Autodesk Fusion 360 part; units mm, degrees
(part 29 of 40)
  spline S86 degree 5 poles (187.9372, 93.9655) (187.9249, 93.9372) (187.9012, 93.8802) (187.868, 93.7938) (187.8281, 93.6771) (187.7842, 93.5289) (187.7447, 93.3792) (187.7079, 93.2286) (187.6725, 93.0774) (187.638, 92.9259) (187.6046, 92.774) (187.5726, 92.6217) (187.5424, 92.4688) (187.5144, 92.3152) (187.4885, 92.1609) (187.4646, 92.006) (187.4423, 91.8506) (187.4215, 91.6948) (187.4019, 91.5386) (187.3835, 91.3821) (187.3662, 91.2253) (187.3502, 91.0682) (187.3355, 90.9107) (187.3222, 90.7529) (187.3102, 90.5947) (187.2995, 90.4362) (187.29, 90.2774) (187.2816, 90.1183) (187.2743, 89.9589) (187.2682, 89.7993) (187.2631, 89.6395) (187.2591, 89.4794) (187.2563, 89.3191) (187.2544, 89.1585) (187.2537, 88.9977) (187.254, 88.8367) (187.2554, 88.6755) (187.2578, 88.5141) (187.2612, 88.3525) (187.2655, 88.1907) (187.2709, 88.0288) (187.2772, 87.8666) (187.2845, 87.7043) (187.2928, 87.5419) (187.302, 87.3793) (187.3121, 87.2165) (187.3232, 87.0536) (187.3353, 86.8905) (187.3482, 86.7273) (187.362, 86.564) (187.3768, 86.4005) (187.3924, 86.2369) (187.409, 86.0732) (187.4264, 85.9094) (187.4447, 85.7455) (187.4639, 85.5815) (187.484, 85.4174) (187.5049, 85.2532) (187.5266, 85.0889) (187.5492, 84.9245) (187.5727, 84.76) (187.597, 84.5954) (187.6222, 84.4308) (187.6481, 84.266) (187.6749, 84.1013) (187.7026, 83.9364) (187.731, 83.7715) (187.7602, 83.6065) (187.7903, 83.4415) (187.8212, 83.2764) (187.8528, 83.1113) (187.8788, 82.9792) (187.8986, 82.8801) (187.912, 82.814) (187.9188, 82.7809) knots 0 0 0 0 0 0 0.01428571 0.02857143 0.04285714 0.05714286 0.07142857 0.08571429 0.1 0.11428571 0.12857143 0.14285714 0.15714286 0.17142857 0.18571429 0.2 0.21428571 0.22857143 0.24285714 0.25714286 0.27142857 0.28571429 0.3 0.31428571 0.32857143 0.34285714 0.35714286 0.37142857 0.38571429 0.4 0.41428571 0.42857143 0.44285714 0.45714286 0.47142857 0.48571429 0.5 0.51428571 0.52857143 0.54285714 0.55714286 0.57142857 0.58571429 0.6 0.61428571 0.62857143 0.64285714 0.65714286 0.67142857 0.68571429 0.7 0.71428571 0.72857143 0.74285714 0.75714286 0.77142857 0.78571429 0.8 0.81428571 0.82857143 0.84285714 0.85714286 0.87142857 0.88571429 0.9 0.91428571 0.92857143 0.94285714 0.95714286 0.97142857 0.98571429 1 1 1 1 1 1
  line L6451 (187.9372, 93.9655) -> (187.9249, 93.9372) construction
  line L6452 (187.9249, 93.9372) -> (187.9012, 93.8802) construction
  line L6453 (187.9012, 93.8802) -> (187.868, 93.7938) construction
  line L6454 (187.868, 93.7938) -> (187.8281, 93.6771) construction
  line L6455 (187.8281, 93.6771) -> (187.7842, 93.5289) construction
  line L6456 (187.7842, 93.5289) -> (187.7447, 93.3792) construction
  line L6457 (187.7447, 93.3792) -> (187.7079, 93.2286) construction
  line L6458 (187.7079, 93.2286) -> (187.6725, 93.0774) construction
  line L6459 (187.6725, 93.0774) -> (187.638, 92.9259) construction
  line L6460 (187.638, 92.9259) -> (187.6046, 92.774) construction
  line L6461 (187.6046, 92.774) -> (187.5726, 92.6217) construction
  line L6462 (187.5726, 92.6217) -> (187.5424, 92.4688) construction
  line L6463 (187.5424, 92.4688) -> (187.5144, 92.3152) construction
  line L6464 (187.5144, 92.3152) -> (187.4885, 92.1609) construction
  line L6465 (187.4885, 92.1609) -> (187.4646, 92.006) construction
  line L6466 (187.4646, 92.006) -> (187.4423, 91.8506) construction
  line L6467 (187.4423, 91.8506) -> (187.4215, 91.6948) construction
  line L6468 (187.4215, 91.6948) -> (187.4019, 91.5386) construction
  line L6469 (187.4019, 91.5386) -> (187.3835, 91.3821) construction
  line L6470 (187.3835, 91.3821) -> (187.3662, 91.2253) construction
  line L6471 (187.3662, 91.2253) -> (187.3502, 91.0682) construction
  line L6472 (187.3502, 91.0682) -> (187.3355, 90.9107) construction
  line L6473 (187.3355, 90.9107) -> (187.3222, 90.7529) construction
  line L6474 (187.3222, 90.7529) -> (187.3102, 90.5947) construction
  line L6475 (187.3102, 90.5947) -> (187.2995, 90.4362) construction
  line L6476 (187.2995, 90.4362) -> (187.29, 90.2774) construction
  line L6477 (187.29, 90.2774) -> (187.2816, 90.1183) construction
  line L6478 (187.2816, 90.1183) -> (187.2743, 89.9589) construction
  line L6479 (187.2743, 89.9589) -> (187.2682, 89.7993) construction
  line L6480 (187.2682, 89.7993) -> (187.2631, 89.6395) construction
  line L6481 (187.2631, 89.6395) -> (187.2591, 89.4794) construction
  line L6482 (187.2591, 89.4794) -> (187.2563, 89.3191) construction
  line L6483 (187.2563, 89.3191) -> (187.2544, 89.1585) construction
  line L6484 (187.2544, 89.1585) -> (187.2537, 88.9977) construction
  line L6485 (187.2537, 88.9977) -> (187.254, 88.8367) construction
  line L6486 (187.254, 88.8367) -> (187.2554, 88.6755) construction
  line L6487 (187.2554, 88.6755) -> (187.2578, 88.5141) construction
  line L6488 (187.2578, 88.5141) -> (187.2612, 88.3525) construction
  line L6489 (187.2612, 88.3525) -> (187.2655, 88.1907) construction
  line L6490 (187.2655, 88.1907) -> (187.2709, 88.0288) construction
  line L6491 (187.2709, 88.0288) -> (187.2772, 87.8666) construction
  line L6492 (187.2772, 87.8666) -> (187.2845, 87.7043) construction
  line L6493 (187.2845, 87.7043) -> (187.2928, 87.5419) construction
  line L6494 (187.2928, 87.5419) -> (187.302, 87.3793) construction
  line L6495 (187.302, 87.3793) -> (187.3121, 87.2165) construction
  line L6496 (187.3121, 87.2165) -> (187.3232, 87.0536) construction
  line L6497 (187.3232, 87.0536) -> (187.3353, 86.8905) construction
  line L6498 (187.3353, 86.8905) -> (187.3482, 86.7273) construction
  line L6499 (187.3482, 86.7273) -> (187.362, 86.564) construction
  line L6500 (187.362, 86.564) -> (187.3768, 86.4005) construction
  line L6501 (187.3768, 86.4005) -> (187.3924, 86.2369) construction
  line L6502 (187.3924, 86.2369) -> (187.409, 86.0732) construction
  line L6503 (187.409, 86.0732) -> (187.4264, 85.9094) construction
  line L6504 (187.4264, 85.9094) -> (187.4447, 85.7455) construction
  line L6505 (187.4447, 85.7455) -> (187.4639, 85.5815) construction
  line L6506 (187.4639, 85.5815) -> (187.484, 85.4174) construction
  line L6507 (187.484, 85.4174) -> (187.5049, 85.2532) construction
  line L6508 (187.5049, 85.2532) -> (187.5266, 85.0889) construction
  line L6509 (187.5266, 85.0889) -> (187.5492, 84.9245) construction
  line L6510 (187.5492, 84.9245) -> (187.5727, 84.76) construction
  line L6511 (187.5727, 84.76) -> (187.597, 84.5954) construction
  line L6512 (187.597, 84.5954) -> (187.6222, 84.4308) construction
  line L6513 (187.6222, 84.4308) -> (187.6481, 84.266) construction
  line L6514 (187.6481, 84.266) -> (187.6749, 84.1013) construction
  line L6515 (187.6749, 84.1013) -> (187.7026, 83.9364) construction
  line L6516 (187.7026, 83.9364) -> (187.731, 83.7715) construction
  line L6517 (187.731, 83.7715) -> (187.7602, 83.6065) construction
  line L6518 (187.7602, 83.6065) -> (187.7903, 83.4415) construction
  line L6519 (187.7903, 83.4415) -> (187.8212, 83.2764) construction
  line L6520 (187.8212, 83.2764) -> (187.8528, 83.1113) construction
  line L6521 (187.8528, 83.1113) -> (187.8788, 82.9792) construction
  line L6522 (187.8788, 82.9792) -> (187.8986, 82.8801) construction
  line L6523 (187.8986, 82.8801) -> (187.912, 82.814) construction
  line L6524 (187.912, 82.814) -> (187.9188, 82.7809) construction
  line L6525 (152.9878, 155.5428) -> (151.3635, 155.6951)
  line L6526 (199.127, 207.9623) -> (198.7698, 209.5542)
  line L6527 (225.137, 207.9623) -> (225.4942, 209.5542)
  line L6528 (217.6748, 209.1442) -> (217.8271, 210.7685)
  line L6529 (251.3803, 194.5906) -> (252.4583, 195.8153)
  line L6530 (271.2762, 155.5428) -> (272.9005, 155.6951)
  line L6531 (172.8837, 194.5906) -> (171.8057, 195.8153)
  line L6532 (181.8522, 201.1066) -> (181.0205, 202.5103)
  line L6533 (157.5954, 173.5481) -> (156.0975, 174.1948)
  line L6534 (167.5414, 189.2483) -> (166.3167, 190.3263)
  spline S87 degree 5 poles (166.3167, 109.6737) (166.2935, 109.6533) (166.2466, 109.6132) (166.1747, 109.5549) (166.076, 109.4808) (165.9487, 109.3934) (165.8185, 109.3096) (165.6866, 109.228) (165.5538, 109.1476) (165.4203, 109.068) (165.2862, 108.9893) (165.1513, 108.9117) (165.0152, 108.8358) (164.8777, 108.7617) (164.739, 108.6894) (164.5991, 108.6187) (164.4582, 108.5496) (164.3164, 108.4816) (164.1739, 108.4147) (164.0308, 108.3488) (163.887, 108.284) (163.7425, 108.2202) (163.5973, 108.1576) (163.4513, 108.0961) (163.3046, 108.0358) (163.1571, 107.9766) (163.009, 107.9185) (162.8603, 107.8614) (162.711, 107.8053) (162.5611, 107.7501) (162.4106, 107.6959) (162.2596, 107.6426) (162.108, 107.5903) (161.9559, 107.539) (161.8032, 107.4886) (161.65, 107.4392) (161.4962, 107.3906) (161.342, 107.343) (161.1873, 107.2963) (161.0321, 107.2505) (160.8764, 107.2055) (160.7202, 107.1614) (160.5636, 107.1182) (160.4065, 107.0759) (160.249, 107.0344) (160.0911, 106.9937) (159.9327, 106.9539) (159.7739, 106.915) (159.6147, 106.8769) (159.4551, 106.8396) (159.2951, 106.8031) (159.1347, 106.7674) (158.9739, 106.7326) (158.8127, 106.6985) (158.6511, 106.6653) (158.4892, 106.6328) (158.3269, 106.6012) (158.1643, 106.5703) (158.0013, 106.5403) (157.838, 106.511) (157.6743, 106.4825) (157.5103, 106.4547) (157.3459, 106.4277) (157.1812, 106.4016) (157.0162, 106.3761) (156.8509, 106.3514) (156.6853, 106.3275) (156.5194, 106.3044) (156.3531, 106.282) (156.1866, 106.2603) (156.0198, 106.2394) (155.8861, 106.2233) (155.7857, 106.2115) (155.7187, 106.2038) (155.6851, 106.2) knots 0 0 0 0 0 0 0.01428571 0.02857143 0.04285714 0.05714286 0.07142857 0.08571429 0.1 0.11428571 0.12857143 0.14285714 0.15714286 0.17142857 0.18571429 0.2 0.21428571 0.22857143 0.24285714 0.25714286 0.27142857 0.28571429 0.3 0.31428571 0.32857143 0.34285714 0.35714286 0.37142857 0.38571429 0.4 0.41428571 0.42857143 0.44285714 0.45714286 0.47142857 0.48571429 0.5 0.51428571 0.52857143 0.54285714 0.55714286 0.57142857 0.58571429 0.6 0.61428571 0.62857143 0.64285714 0.65714286 0.67142857 0.68571429 0.7 0.71428571 0.72857143 0.74285714 0.75714286 0.77142857 0.78571429 0.8 0.81428571 0.82857143 0.84285714 0.85714286 0.87142857 0.88571429 0.9 0.91428571 0.92857143 0.94285714 0.95714286 0.97142857 0.98571429 1 1 1 1 1 1
  line L6535 (166.3167, 109.6737) -> (166.2935, 109.6533) construction
  line L6536 (166.2935, 109.6533) -> (166.2466, 109.6132) construction
  line L6537 (166.2466, 109.6132) -> (166.1747, 109.5549) construction
  line L6538 (166.1747, 109.5549) -> (166.076, 109.4808) construction
  line L6539 (166.076, 109.4808) -> (165.9487, 109.3934) construction
  line L6540 (165.9487, 109.3934) -> (165.8185, 109.3096) construction
  line L6541 (165.8185, 109.3096) -> (165.6866, 109.228) construction
  line L6542 (165.6866, 109.228) -> (165.5538, 109.1476) construction
  line L6543 (165.5538, 109.1476) -> (165.4203, 109.068) construction
  line L6544 (165.4203, 109.068) -> (165.2862, 108.9893) construction
  line L6545 (165.2862, 108.9893) -> (165.1513, 108.9117) construction
  line L6546 (165.1513, 108.9117) -> (165.0152, 108.8358) construction
  line L6547 (165.0152, 108.8358) -> (164.8777, 108.7617) construction
  line L6548 (164.8777, 108.7617) -> (164.739, 108.6894) construction
  line L6549 (164.739, 108.6894) -> (164.5991, 108.6187) construction
  line L6550 (164.5991, 108.6187) -> (164.4582, 108.5496) construction
  line L6551 (164.4582, 108.5496) -> (164.3164, 108.4816) construction
  line L6552 (164.3164, 108.4816) -> (164.1739, 108.4147) construction
  line L6553 (164.1739, 108.4147) -> (164.0308, 108.3488) construction
  line L6554 (164.0308, 108.3488) -> (163.887, 108.284) construction
  line L6555 (163.887, 108.284) -> (163.7425, 108.2202) construction
  line L6556 (163.7425, 108.2202) -> (163.5973, 108.1576) construction
  line L6557 (163.5973, 108.1576) -> (163.4513, 108.0961) construction
  line L6558 (163.4513, 108.0961) -> (163.3046, 108.0358) construction
  line L6559 (163.3046, 108.0358) -> (163.1571, 107.9766) construction
  line L6560 (163.1571, 107.9766) -> (163.009, 107.9185) construction
  line L6561 (163.009, 107.9185) -> (162.8603, 107.8614) construction
  line L6562 (162.8603, 107.8614) -> (162.711, 107.8053) construction
  line L6563 (162.711, 107.8053) -> (162.5611, 107.7501) construction
  line L6564 (162.5611, 107.7501) -> (162.4106, 107.6959) construction
  line L6565 (162.4106, 107.6959) -> (162.2596, 107.6426) construction
  line L6566 (162.2596, 107.6426) -> (162.108, 107.5903) construction
  line L6567 (162.108, 107.5903) -> (161.9559, 107.539) construction
  line L6568 (161.9559, 107.539) -> (161.8032, 107.4886) construction
  line L6569 (161.8032, 107.4886) -> (161.65, 107.4392) construction
  line L6570 (161.65, 107.4392) -> (161.4962, 107.3906) construction
  line L6571 (161.4962, 107.3906) -> (161.342, 107.343) construction
  line L6572 (161.342, 107.343) -> (161.1873, 107.2963) construction
  line L6573 (161.1873, 107.2963) -> (161.0321, 107.2505) construction
  line L6574 (161.0321, 107.2505) -> (160.8764, 107.2055) construction
  line L6575 (160.8764, 107.2055) -> (160.7202, 107.1614) construction
  line L6576 (160.7202, 107.1614) -> (160.5636, 107.1182) construction
  line L6577 (160.5636, 107.1182) -> (160.4065, 107.0759) construction
  line L6578 (160.4065, 107.0759) -> (160.249, 107.0344) construction
  line L6579 (160.249, 107.0344) -> (160.0911, 106.9937) construction
  line L6580 (160.0911, 106.9937) -> (159.9327, 106.9539) construction
  line L6581 (159.9327, 106.9539) -> (159.7739, 106.915) construction
  line L6582 (159.7739, 106.915) -> (159.6147, 106.8769) construction
  line L6583 (159.6147, 106.8769) -> (159.4551, 106.8396) construction
  line L6584 (159.4551, 106.8396) -> (159.2951, 106.8031) construction
  line L6585 (159.2951, 106.8031) -> (159.1347, 106.7674) construction
  line L6586 (159.1347, 106.7674) -> (158.9739, 106.7326) construction
  line L6587 (158.9739, 106.7326) -> (158.8127, 106.6985) construction
  line L6588 (158.8127, 106.6985) -> (158.6511, 106.6653) construction
  line L6589 (158.6511, 106.6653) -> (158.4892, 106.6328) construction
  line L6590 (158.4892, 106.6328) -> (158.3269, 106.6012) construction
  line L6591 (158.3269, 106.6012) -> (158.1643, 106.5703) construction
  line L6592 (158.1643, 106.5703) -> (158.0013, 106.5403) construction
  line L6593 (158.0013, 106.5403) -> (157.838, 106.511) construction
  line L6594 (157.838, 106.511) -> (157.6743, 106.4825) construction
  line L6595 (157.6743, 106.4825) -> (157.5103, 106.4547) construction
  line L6596 (157.5103, 106.4547) -> (157.3459, 106.4277) construction
  line L6597 (157.3459, 106.4277) -> (157.1812, 106.4016) construction
  line L6598 (157.1812, 106.4016) -> (157.0162, 106.3761) construction
  line L6599 (157.0162, 106.3761) -> (156.8509, 106.3514) construction
  line L6600 (156.8509, 106.3514) -> (156.6853, 106.3275) construction
  line L6601 (156.6853, 106.3275) -> (156.5194, 106.3044) construction
  line L6602 (156.5194, 106.3044) -> (156.3531, 106.282) construction
  line L6603 (156.3531, 106.282) -> (156.1866, 106.2603) construction
  line L6604 (156.1866, 106.2603) -> (156.0198, 106.2394) construction
  line L6605 (156.0198, 106.2394) -> (155.8861, 106.2233) construction
  line L6606 (155.8861, 106.2233) -> (155.7857, 106.2115) construction
  line L6607 (155.7857, 106.2115) -> (155.7187, 106.2038) construction
  line L6608 (155.7187, 106.2038) -> (155.6851, 106.2) construction
  arc A175 (236.3452, 217.2191) -> (232.0535, 218.6136) centre (212.132, 150) ccw
  spline S88 degree 5 poles (236.3268, 206.0345) (236.3391, 206.0628) (236.3628, 206.1198) (236.396, 206.2062) (236.4359, 206.3229) (236.4798, 206.4711) (236.5193, 206.6208) (236.5561, 206.7714) (236.5915, 206.9226) (236.626, 207.0741) (236.6594, 207.226) (236.6914, 207.3783) (236.7216, 207.5312) (236.7496, 207.6848) (236.7755, 207.8391) (236.7994, 207.994) (236.8217, 208.1494) (236.8425, 208.3052) (236.8621, 208.4614) (236.8805, 208.6179) (236.8978, 208.7747) (236.9138, 208.9318) (236.9285, 209.0893) (236.9418, 209.2471) (236.9538, 209.4053) (236.9645, 209.5638) (236.974, 209.7226) (236.9824, 209.8817) (236.9897, 210.0411) (236.9958, 210.2007) (237.0009, 210.3605) (237.0049, 210.5206) (237.0077, 210.6809) (237.0096, 210.8415) (237.0103, 211.0023) (237.01, 211.1633) (237.0086, 211.3245) (237.0062, 211.4859) (237.0028, 211.6475) (236.9985, 211.8093) (236.9931, 211.9712) (236.9868, 212.1334) (236.9795, 212.2957) (236.9712, 212.4581) (236.962, 212.6207) (236.9519, 212.7835) (236.9408, 212.9464) (236.9287, 213.1095) (236.9158, 213.2727) (236.902, 213.436) (236.8872, 213.5995) (236.8716, 213.7631) (236.855, 213.9268) (236.8376, 214.0906) (236.8193, 214.2545) (236.8001, 214.4185) (236.78, 214.5826) (236.7591, 214.7468) (236.7374, 214.9111) (236.7148, 215.0755) (236.6913, 215.24) (236.667, 215.4046) (236.6418, 215.5692) (236.6159, 215.734) (236.5891, 215.8987) (236.5614, 216.0636) (236.533, 216.2285) (236.5038, 216.3935) (236.4737, 216.5585) (236.4428, 216.7236) (236.4112, 216.8887) (236.3852, 217.0208) (236.3654, 217.1199) (236.352, 217.186) (236.3452, 217.2191) knots 0 0 0 0 0 0 0.01428571 0.02857143 0.04285714 0.05714286 0.07142857 0.08571429 0.1 0.11428571 0.12857143 0.14285714 0.15714286 0.17142857 0.18571429 0.2 0.21428571 0.22857143 0.24285714 0.25714286 0.27142857 0.28571429 0.3 0.31428571 0.32857143 0.34285714 0.35714286 0.37142857 0.38571429 0.4 0.41428571 0.42857143 0.44285714 0.45714286 0.47142857 0.48571429 0.5 0.51428571 0.52857143 0.54285714 0.55714286 0.57142857 0.58571429 0.6 0.61428571 0.62857143 0.64285714 0.65714286 0.67142857 0.68571429 0.7 0.71428571 0.72857143 0.74285714 0.75714286 0.77142857 0.78571429 0.8 0.81428571 0.82857143 0.84285714 0.85714286 0.87142857 0.88571429 0.9 0.91428571 0.92857143 0.94285714 0.95714286 0.97142857 0.98571429 1 1 1 1 1 1
  line L6609 (236.3268, 206.0345) -> (236.3391, 206.0628) construction
  line L6610 (236.3391, 206.0628) -> (236.3628, 206.1198) construction
  line L6611 (236.3628, 206.1198) -> (236.396, 206.2062) construction
  line L6612 (236.396, 206.2062) -> (236.4359, 206.3229) construction
  line L6613 (236.4359, 206.3229) -> (236.4798, 206.4711) construction
  line L6614 (236.4798, 206.4711) -> (236.5193, 206.6208) construction
  line L6615 (236.5193, 206.6208) -> (236.5561, 206.7714) construction
  line L6616 (236.5561, 206.7714) -> (236.5915, 206.9226) construction
  line L6617 (236.5915, 206.9226) -> (236.626, 207.0741) construction
  line L6618 (236.626, 207.0741) -> (236.6594, 207.226) construction
  line L6619 (236.6594, 207.226) -> (236.6914, 207.3783) construction
  line L6620 (236.6914, 207.3783) -> (236.7216, 207.5312) construction
  line L6621 (236.7216, 207.5312) -> (236.7496, 207.6848) construction
  line L6622 (236.7496, 207.6848) -> (236.7755, 207.8391) construction
  line L6623 (236.7755, 207.8391) -> (236.7994, 207.994) construction
  line L6624 (236.7994, 207.994) -> (236.8217, 208.1494) construction
  line L6625 (236.8217, 208.1494) -> (236.8425, 208.3052) construction
  line L6626 (236.8425, 208.3052) -> (236.8621, 208.4614) construction
  line L6627 (236.8621, 208.4614) -> (236.8805, 208.6179) construction
  line L6628 (236.8805, 208.6179) -> (236.8978, 208.7747) construction
  line L6629 (236.8978, 208.7747) -> (236.9138, 208.9318) construction
  line L6630 (236.9138, 208.9318) -> (236.9285, 209.0893) construction
  line L6631 (236.9285, 209.0893) -> (236.9418, 209.2471) construction
  line L6632 (236.9418, 209.2471) -> (236.9538, 209.4053) construction
  line L6633 (236.9538, 209.4053) -> (236.9645, 209.5638) construction
  line L6634 (236.9645, 209.5638) -> (236.974, 209.7226) construction
  line L6635 (236.974, 209.7226) -> (236.9824, 209.8817) construction
  line L6636 (236.9824, 209.8817) -> (236.9897, 210.0411) construction
  line L6637 (236.9897, 210.0411) -> (236.9958, 210.2007) construction
  line L6638 (236.9958, 210.2007) -> (237.0009, 210.3605) construction
  line L6639 (237.0009, 210.3605) -> (237.0049, 210.5206) construction
  line L6640 (237.0049, 210.5206) -> (237.0077, 210.6809) construction
  line L6641 (237.0077, 210.6809) -> (237.0096, 210.8415) construction
  line L6642 (237.0096, 210.8415) -> (237.0103, 211.0023) construction
  line L6643 (237.0103, 211.0023) -> (237.01, 211.1633) construction
  line L6644 (237.01, 211.1633) -> (237.0086, 211.3245) construction
  line L6645 (237.0086, 211.3245) -> (237.0062, 211.4859) construction
  line L6646 (237.0062, 211.4859) -> (237.0028, 211.6475) construction
  line L6647 (237.0028, 211.6475) -> (236.9985, 211.8093) construction
  line L6648 (236.9985, 211.8093) -> (236.9931, 211.9712) construction
  line L6649 (236.9931, 211.9712) -> (236.9868, 212.1334) construction
  line L6650 (236.9868, 212.1334) -> (236.9795, 212.2957) construction
  line L6651 (236.9795, 212.2957) -> (236.9712, 212.4581) construction
  line L6652 (236.9712, 212.4581) -> (236.962, 212.6207) construction
  line L6653 (236.962, 212.6207) -> (236.9519, 212.7835) construction
  line L6654 (236.9519, 212.7835) -> (236.9408, 212.9464) construction
  line L6655 (236.9408, 212.9464) -> (236.9287, 213.1095) construction
  line L6656 (236.9287, 213.1095) -> (236.9158, 213.2727) construction
  line L6657 (236.9158, 213.2727) -> (236.902, 213.436) construction
  line L6658 (236.902, 213.436) -> (236.8872, 213.5995) construction
  line L6659 (236.8872, 213.5995) -> (236.8716, 213.7631) construction
  line L6660 (236.8716, 213.7631) -> (236.855, 213.9268) construction
  line L6661 (236.855, 213.9268) -> (236.8376, 214.0906) construction
  line L6662 (236.8376, 214.0906) -> (236.8193, 214.2545) construction
  line L6663 (236.8193, 214.2545) -> (236.8001, 214.4185) construction
  line L6664 (236.8001, 214.4185) -> (236.78, 214.5826) construction
  line L6665 (236.78, 214.5826) -> (236.7591, 214.7468) construction
  line L6666 (236.7591, 214.7468) -> (236.7374, 214.9111) construction
  line L6667 (236.7374, 214.9111) -> (236.7148, 215.0755) construction
  line L6668 (236.7148, 215.0755) -> (236.6913, 215.24) construction
  line L6669 (236.6913, 215.24) -> (236.667, 215.4046) construction
  line L6670 (236.667, 215.4046) -> (236.6418, 215.5692) construction
  line L6671 (236.6418, 215.5692) -> (236.6159, 215.734) construction
  line L6672 (236.6159, 215.734) -> (236.5891, 215.8987) construction
  line L6673 (236.5891, 215.8987) -> (236.5614, 216.0636) construction
  line L6674 (236.5614, 216.0636) -> (236.533, 216.2285) construction
  line L6675 (236.533, 216.2285) -> (236.5038, 216.3935) construction
  line L6676 (236.5038, 216.3935) -> (236.4737, 216.5585) construction
  line L6677 (236.4737, 216.5585) -> (236.4428, 216.7236) construction
  line L6678 (236.4428, 216.7236) -> (236.4112, 216.8887) construction
  line L6679 (236.4112, 216.8887) -> (236.3852, 217.0208) construction
  line L6680 (236.3852, 217.0208) -> (236.3654, 217.1199) construction
  line L6681 (236.3654, 217.1199) -> (236.352, 217.186) construction
  line L6682 (236.352, 217.186) -> (236.3452, 217.2191) construction
  arc A176 (239.7302, 200.3721) -> (242.4118, 201.1066) centre (240.6912, 202.1261) ccw
  spline S89 degree 5 poles (271.6862, 136.6378) (271.7163, 136.631) (271.7764, 136.6167) (271.8658, 136.5929) (271.9837, 136.5565) (272.1293, 136.5049) (272.2736, 136.4489) (272.4172, 136.3901) (272.5603, 136.3299) (272.7031, 136.2687) (272.8456, 136.2065) (272.9877, 136.1429) (273.1291, 136.0774) (273.2699, 136.0098) (273.4099, 135.94) (273.5493, 135.8684) (273.6881, 135.795) (273.8264, 135.7203) (273.9642, 135.6443) (274.1017, 135.5673) (274.2387, 135.4891) (274.3752, 135.4096) (274.5112, 135.3289) (274.6468, 135.247) (274.7818, 135.1637) (274.9163, 135.0792) (275.0504, 134.9936) (275.184, 134.9068) (275.3172, 134.819) (275.45, 134.7302) (275.5823, 134.6403) (275.7141, 134.5494) (275.8455, 134.4575) (275.9765, 134.3646) (276.107, 134.2707) (276.237, 134.1758) (276.3666, 134.08) (276.4958, 133.9832) (276.6246, 133.8854) (276.7529, 133.7868) (276.8808, 133.6873) (277.0082, 133.5869) (277.1352, 133.4856) (277.2618, 133.3834) (277.388, 133.2804) (277.5137, 133.1765) (277.639, 133.0717) (277.7638, 132.9662) (277.8882, 132.8598) (278.0122, 132.7526) (278.1358, 132.6445) (278.2589, 132.5357) (278.3817, 132.4261) (278.5039, 132.3158) (278.6258, 132.2046) (278.7472, 132.0927) (278.8682, 131.98) (278.9888, 131.8665) (279.1089, 131.7523) (279.2286, 131.6374) (279.3479, 131.5218) (279.4667, 131.4054) (279.5851, 131.2882) (279.7031, 131.1704) (279.8207, 131.0519) (279.9378, 130.9326) (280.0545, 130.8127) (280.1708, 130.6921) (280.2866, 130.5707) (280.402, 130.4488) (280.517, 130.3261) (280.6087, 130.2274) (280.6772, 130.1531) (280.7228, 130.1034) (280.7456, 130.0785) knots 0 0 0 0 0 0 0.01428571 0.02857143 0.04285714 0.05714286 0.07142857 0.08571429 0.1 0.11428571 0.12857143 0.14285714 0.15714286 0.17142857 0.18571429 0.2 0.21428571 0.22857143 0.24285714 0.25714286 0.27142857 0.28571429 0.3 0.31428571 0.32857143 0.34285714 0.35714286 0.37142857 0.38571429 0.4 0.41428571 0.42857143 0.44285714 0.45714286 0.47142857 0.48571429 0.5 0.51428571 0.52857143 0.54285714 0.55714286 0.57142857 0.58571429 0.6 0.61428571 0.62857143 0.64285714 0.65714286 0.67142857 0.68571429 0.7 0.71428571 0.72857143 0.74285714 0.75714286 0.77142857 0.78571429 0.8 0.81428571 0.82857143 0.84285714 0.85714286 0.87142857 0.88571429 0.9 0.91428571 0.92857143 0.94285714 0.95714286 0.97142857 0.98571429 1 1 1 1 1 1
  line L6683 (271.6862, 136.6378) -> (271.7163, 136.631) construction
  line L6684 (271.7163, 136.631) -> (271.7764, 136.6167) construction
  line L6685 (271.7764, 136.6167) -> (271.8658, 136.5929) construction
  line L6686 (271.8658, 136.5929) -> (271.9837, 136.5565) construction
  line L6687 (271.9837, 136.5565) -> (272.1293, 136.5049) construction
  line L6688 (272.1293, 136.5049) -> (272.2736, 136.4489) construction
  line L6689 (272.2736, 136.4489) -> (272.4172, 136.3901) construction
  line L6690 (272.4172, 136.3901) -> (272.5603, 136.3299) construction
  line L6691 (272.5603, 136.3299) -> (272.7031, 136.2687) construction
  line L6692 (272.7031, 136.2687) -> (272.8456, 136.2065) construction
  line L6693 (272.8456, 136.2065) -> (272.9877, 136.1429) construction
  line L6694 (272.9877, 136.1429) -> (273.1291, 136.0774) construction
  line L6695 (273.1291, 136.0774) -> (273.2699, 136.0098) construction
  line L6696 (273.2699, 136.0098) -> (273.4099, 135.94) construction
  line L6697 (273.4099, 135.94) -> (273.5493, 135.8684) construction
  line L6698 (273.5493, 135.8684) -> (273.6881, 135.795) construction
  line L6699 (273.6881, 135.795) -> (273.8264, 135.7203) construction
  line L6700 (273.8264, 135.7203) -> (273.9642, 135.6443) construction
  line L6701 (273.9642, 135.6443) -> (274.1017, 135.5673) construction
  line L6702 (274.1017, 135.5673) -> (274.2387, 135.4891) construction
  line L6703 (274.2387, 135.4891) -> (274.3752, 135.4096) construction
  line L6704 (274.3752, 135.4096) -> (274.5112, 135.3289) construction
  line L6705 (274.5112, 135.3289) -> (274.6468, 135.247) construction
  line L6706 (274.6468, 135.247) -> (274.7818, 135.1637) construction
  line L6707 (274.7818, 135.1637) -> (274.9163, 135.0792) construction
  line L6708 (274.9163, 135.0792) -> (275.0504, 134.9936) construction
  line L6709 (275.0504, 134.9936) -> (275.184, 134.9068) construction
  line L6710 (275.184, 134.9068) -> (275.3172, 134.819) construction
  line L6711 (275.3172, 134.819) -> (275.45, 134.7302) construction
  line L6712 (275.45, 134.7302) -> (275.5823, 134.6403) construction
  line L6713 (275.5823, 134.6403) -> (275.7141, 134.5494) construction
  line L6714 (275.7141, 134.5494) -> (275.8455, 134.4575) construction
  line L6715 (275.8455, 134.4575) -> (275.9765, 134.3646) construction
  line L6716 (275.9765, 134.3646) -> (276.107, 134.2707) construction
  line L6717 (276.107, 134.2707) -> (276.237, 134.1758) construction
  line L6718 (276.237, 134.1758) -> (276.3666, 134.08) construction
  line L6719 (276.3666, 134.08) -> (276.4958, 133.9832) construction
  line L6720 (276.4958, 133.9832) -> (276.6246, 133.8854) construction
  line L6721 (276.6246, 133.8854) -> (276.7529, 133.7868) construction
  line L6722 (276.7529, 133.7868) -> (276.8808, 133.6873) construction
  line L6723 (276.8808, 133.6873) -> (277.0082, 133.5869) construction
  line L6724 (277.0082, 133.5869) -> (277.1352, 133.4856) construction
  line L6725 (277.1352, 133.4856) -> (277.2618, 133.3834) construction
  line L6726 (277.2618, 133.3834) -> (277.388, 133.2804) construction
  line L6727 (277.388, 133.2804) -> (277.5137, 133.1765) construction
  line L6728 (277.5137, 133.1765) -> (277.639, 133.0717) construction
  line L6729 (277.639, 133.0717) -> (277.7638, 132.9662) construction
  line L6730 (277.7638, 132.9662) -> (277.8882, 132.8598) construction
  line L6731 (277.8882, 132.8598) -> (278.0122, 132.7526) construction
  line L6732 (278.0122, 132.7526) -> (278.1358, 132.6445) construction
  line L6733 (278.1358, 132.6445) -> (278.2589, 132.5357) construction
  line L6734 (278.2589, 132.5357) -> (278.3817, 132.4261) construction
  line L6735 (278.3817, 132.4261) -> (278.5039, 132.3158) construction
  line L6736 (278.5039, 132.3158) -> (278.6258, 132.2046) construction
  line L6737 (278.6258, 132.2046) -> (278.7472, 132.0927) construction
  line L6738 (278.7472, 132.0927) -> (278.8682, 131.98) construction
  line L6739 (278.8682, 131.98) -> (278.9888, 131.8665) construction
  line L6740 (278.9888, 131.8665) -> (279.1089, 131.7523) construction
  line L6741 (279.1089, 131.7523) -> (279.2286, 131.6374) construction
  line L6742 (279.2286, 131.6374) -> (279.3479, 131.5218) construction
  line L6743 (279.3479, 131.5218) -> (279.4667, 131.4054) construction
  line L6744 (279.4667, 131.4054) -> (279.5851, 131.2882) construction
  line L6745 (279.5851, 131.2882) -> (279.7031, 131.1704) construction
  line L6746 (279.7031, 131.1704) -> (279.8207, 131.0519) construction
  line L6747 (279.8207, 131.0519) -> (279.9378, 130.9326) construction
  line L6748 (279.9378, 130.9326) -> (280.0545, 130.8127) construction
  line L6749 (280.0545, 130.8127) -> (280.1708, 130.6921) construction
  line L6750 (280.1708, 130.6921) -> (280.2866, 130.5707) construction
  line L6751 (280.2866, 130.5707) -> (280.402, 130.4488) construction
  line L6752 (280.402, 130.4488) -> (280.517, 130.3261) construction
  line L6753 (280.517, 130.3261) -> (280.6087, 130.2274) construction
  line L6754 (280.6087, 130.2274) -> (280.6772, 130.1531) construction
  line L6755 (280.6772, 130.1531) -> (280.7228, 130.1034) construction
  line L6756 (280.7228, 130.1034) -> (280.7456, 130.0785) construction
  spline S90 degree 5 poles (257.9473, 190.3263) (257.9705, 190.3467) (258.0174, 190.3868) (258.0893, 190.4451) (258.188, 190.5192) (258.3153, 190.6066) (258.4455, 190.6904) (258.5774, 190.772) (258.7102, 190.8524) (258.8437, 190.932) (258.9778, 191.0107) (259.1127, 191.0883) (259.2488, 191.1642) (259.3863, 191.2383) (259.525, 191.3106) (259.6649, 191.3813) (259.8058, 191.4504) (259.9476, 191.5184) (260.0901, 191.5853) (260.2332, 191.6512) (260.377, 191.716) (260.5215, 191.7798) (260.6667, 191.8424) (260.8127, 191.9039) (260.9594, 191.9642) (261.1069, 192.0234) (261.255, 192.0815) (261.4037, 192.1386) (261.553, 192.1947) (261.7029, 192.2499) (261.8534, 192.3041) (262.0044, 192.3574) (262.156, 192.4097) (262.3081, 192.461) (262.4608, 192.5114) (262.614, 192.5608) (262.7678, 192.6094) (262.922, 192.657) (263.0767, 192.7037) (263.2319, 192.7495) (263.3876, 192.7945) (263.5438, 192.8386) (263.7004, 192.8818) (263.8575, 192.9241) (264.015, 192.9656) (264.1729, 193.0063) (264.3313, 193.0461) (264.4901, 193.085) (264.6493, 193.1231) (264.8089, 193.1604) (264.9689, 193.1969) (265.1293, 193.2326) (265.2901, 193.2674) (265.4513, 193.3015) (265.6129, 193.3347) (265.7748, 193.3672) (265.9371, 193.3988) (266.0997, 193.4297) (266.2627, 193.4597) (266.426, 193.489) (266.5897, 193.5175) (266.7537, 193.5453) (266.9181, 193.5723) (267.0828, 193.5984) (267.2478, 193.6239) (267.4131, 193.6486) (267.5787, 193.6725) (267.7446, 193.6956) (267.9109, 193.718) (268.0774, 193.7397) (268.2442, 193.7606) (268.3779, 193.7767) (268.4783, 193.7885) (268.5453, 193.7962) (268.5789, 193.8) knots 0 0 0 0 0 0 0.01428571 0.02857143 0.04285714 0.05714286 0.07142857 0.08571429 0.1 0.11428571 0.12857143 0.14285714 0.15714286 0.17142857 0.18571429 0.2 0.21428571 0.22857143 0.24285714 0.25714286 0.27142857 0.28571429 0.3 0.31428571 0.32857143 0.34285714 0.35714286 0.37142857 0.38571429 0.4 0.41428571 0.42857143 0.44285714 0.45714286 0.47142857 0.48571429 0.5 0.51428571 0.52857143 0.54285714 0.55714286 0.57142857 0.58571429 0.6 0.61428571 0.62857143 0.64285714 0.65714286 0.67142857 0.68571429 0.7 0.71428571 0.72857143 0.74285714 0.75714286 0.77142857 0.78571429 0.8 0.81428571 0.82857143 0.84285714 0.85714286 0.87142857 0.88571429 0.9 0.91428571 0.92857143 0.94285714 0.95714286 0.97142857 0.98571429 1 1 1 1 1 1
  line L6757 (257.9473, 190.3263) -> (257.9705, 190.3467) construction
  line L6758 (257.9705, 190.3467) -> (258.0174, 190.3868) construction
  line L6759 (258.0174, 190.3868) -> (258.0893, 190.4451) construction
  line L6760 (258.0893, 190.4451) -> (258.188, 190.5192) construction
  line L6761 (258.188, 190.5192) -> (258.3153, 190.6066) construction
  line L6762 (258.3153, 190.6066) -> (258.4455, 190.6904) construction
  line L6763 (258.4455, 190.6904) -> (258.5774, 190.772) construction
  line L6764 (258.5774, 190.772) -> (258.7102, 190.8524) construction
  line L6765 (258.7102, 190.8524) -> (258.8437, 190.932) construction
  line L6766 (258.8437, 190.932) -> (258.9778, 191.0107) construction
  line L6767 (258.9778, 191.0107) -> (259.1127, 191.0883) construction
  line L6768 (259.1127, 191.0883) -> (259.2488, 191.1642) construction
  line L6769 (259.2488, 191.1642) -> (259.3863, 191.2383) construction
  line L6770 (259.3863, 191.2383) -> (259.525, 191.3106) construction
  line L6771 (259.525, 191.3106) -> (259.6649, 191.3813) construction
  line L6772 (259.6649, 191.3813) -> (259.8058, 191.4504) construction
  line L6773 (259.8058, 191.4504) -> (259.9476, 191.5184) construction
  line L6774 (259.9476, 191.5184) -> (260.0901, 191.5853) construction
  line L6775 (260.0901, 191.5853) -> (260.2332, 191.6512) construction
  line L6776 (260.2332, 191.6512) -> (260.377, 191.716) construction
  line L6777 (260.377, 191.716) -> (260.5215, 191.7798) construction
  line L6778 (260.5215, 191.7798) -> (260.6667, 191.8424) construction
  line L6779 (260.6667, 191.8424) -> (260.8127, 191.9039) construction
  line L6780 (260.8127, 191.9039) -> (260.9594, 191.9642) construction
  line L6781 (260.9594, 191.9642) -> (261.1069, 192.0234) construction
  line L6782 (261.1069, 192.0234) -> (261.255, 192.0815) construction
  line L6783 (261.255, 192.0815) -> (261.4037, 192.1386) construction
  line L6784 (261.4037, 192.1386) -> (261.553, 192.1947) construction
  line L6785 (261.553, 192.1947) -> (261.7029, 192.2499) construction
  line L6786 (261.7029, 192.2499) -> (261.8534, 192.3041) construction
  line L6787 (261.8534, 192.3041) -> (262.0044, 192.3574) construction
  line L6788 (262.0044, 192.3574) -> (262.156, 192.4097) construction
  line L6789 (262.156, 192.4097) -> (262.3081, 192.461) construction
  line L6790 (262.3081, 192.461) -> (262.4608, 192.5114) construction
  line L6791 (262.4608, 192.5114) -> (262.614, 192.5608) construction
  line L6792 (262.614, 192.5608) -> (262.7678, 192.6094) construction
  line L6793 (262.7678, 192.6094) -> (262.922, 192.657) construction
  line L6794 (262.922, 192.657) -> (263.0767, 192.7037) construction
  line L6795 (263.0767, 192.7037) -> (263.2319, 192.7495) construction
  line L6796 (263.2319, 192.7495) -> (263.3876, 192.7945) construction
  line L6797 (263.3876, 192.7945) -> (263.5438, 192.8386) construction
  line L6798 (263.5438, 192.8386) -> (263.7004, 192.8818) construction
  line L6799 (263.7004, 192.8818) -> (263.8575, 192.9241) construction
  line L6800 (263.8575, 192.9241) -> (264.015, 192.9656) construction
  line L6801 (264.015, 192.9656) -> (264.1729, 193.0063) construction
  line L6802 (264.1729, 193.0063) -> (264.3313, 193.0461) construction
  line L6803 (264.3313, 193.0461) -> (264.4901, 193.085) construction
  line L6804 (264.4901, 193.085) -> (264.6493, 193.1231) construction
  line L6805 (264.6493, 193.1231) -> (264.8089, 193.1604) construction
  line L6806 (264.8089, 193.1604) -> (264.9689, 193.1969) construction
  line L6807 (264.9689, 193.1969) -> (265.1293, 193.2326) construction
  line L6808 (265.1293, 193.2326) -> (265.2901, 193.2674) construction
  line L6809 (265.2901, 193.2674) -> (265.4513, 193.3015) construction
  line L6810 (265.4513, 193.3015) -> (265.6129, 193.3347) construction
  line L6811 (265.6129, 193.3347) -> (265.7748, 193.3672) construction
  line L6812 (265.7748, 193.3672) -> (265.9371, 193.3988) construction
  line L6813 (265.9371, 193.3988) -> (266.0997, 193.4297) construction
  line L6814 (266.0997, 193.4297) -> (266.2627, 193.4597) construction
  line L6815 (266.2627, 193.4597) -> (266.426, 193.489) construction
  line L6816 (266.426, 193.489) -> (266.5897, 193.5175) construction
  line L6817 (266.5897, 193.5175) -> (266.7537, 193.5453) construction
  line L6818 (266.7537, 193.5453) -> (266.9181, 193.5723) construction
  line L6819 (266.9181, 193.5723) -> (267.0828, 193.5984) construction
  line L6820 (267.0828, 193.5984) -> (267.2478, 193.6239) construction
  line L6821 (267.2478, 193.6239) -> (267.4131, 193.6486) construction
  line L6822 (267.4131, 193.6486) -> (267.5787, 193.6725) construction
  line L6823 (267.5787, 193.6725) -> (267.7446, 193.6956) construction
  line L6824 (267.7446, 193.6956) -> (267.9109, 193.718) construction
  line L6825 (267.9109, 193.718) -> (268.0774, 193.7397) construction
  line L6826 (268.0774, 193.7397) -> (268.2442, 193.7606) construction
  line L6827 (268.2442, 193.7606) -> (268.3779, 193.7767) construction
  line L6828 (268.3779, 193.7767) -> (268.4783, 193.7885) construction
  line L6829 (268.4783, 193.7885) -> (268.5453, 193.7962) construction
  line L6830 (268.5453, 193.7962) -> (268.5789, 193.8) construction
  arc A177 (155.1583, 142.7194) -> (152.9878, 144.4572) centre (153.1745, 142.4659) ccw
  arc A178 (167.5414, 189.2483) -> (170.3188, 189.3784) centre (168.8628, 190.7496) ccw
  arc A179 (201.4504, 93.565) -> (204.8514, 93.0263) centre (212.132, 150) ccw
  spline S91 degree 5 poles (268.1665, 125.8052) (268.1948, 125.7929) (268.2518, 125.7692) (268.3382, 125.736) (268.4549, 125.6961) (268.6031, 125.6522) (268.7528, 125.6127) (268.9034, 125.5759) (269.0546, 125.5405) (269.2061, 125.506) (269.358, 125.4726) (269.5103, 125.4406) (269.6632, 125.4104) (269.8168, 125.3824) (269.9711, 125.3565) (270.126, 125.3326) (270.2814, 125.3103) (270.4372, 125.2895) (270.5934, 125.2699) (270.7499, 125.2515) (270.9067, 125.2342) (271.0638, 125.2182) (271.2213, 125.2035) (271.3791, 125.1902) (271.5373, 125.1782) (271.6958, 125.1675) (271.8546, 125.158) (272.0137, 125.1496) (272.1731, 125.1423) (272.3327, 125.1362) (272.4925, 125.1311) (272.6526, 125.1271) (272.8129, 125.1243) (272.9735, 125.1224) (273.1343, 125.1217) (273.2953, 125.122) (273.4565, 125.1234) (273.6179, 125.1258) (273.7795, 125.1292) (273.9413, 125.1335) (274.1032, 125.1389) (274.2654, 125.1452) (274.4277, 125.1525) (274.5901, 125.1608) (274.7527, 125.17) (274.9155, 125.1801) (275.0784, 125.1912) (275.2415, 125.2033) (275.4047, 125.2162) (275.568, 125.23) (275.7315, 125.2448) (275.8951, 125.2604) (276.0588, 125.277) (276.2226, 125.2944) (276.3865, 125.3127) (276.5505, 125.3319) (276.7146, 125.352) (276.8788, 125.3729) (277.0431, 125.3946) (277.2075, 125.4172) (277.372, 125.4407) (277.5366, 125.465) (277.7012, 125.4902) (277.866, 125.5161) (278.0307, 125.5429) (278.1956, 125.5706) (278.3605, 125.599) (278.5255, 125.6282) (278.6905, 125.6583) (278.8556, 125.6892) (279.0207, 125.7208) (279.1528, 125.7468) (279.2519, 125.7666) (279.318, 125.78) (279.3511, 125.7868) knots 0 0 0 0 0 0 0.01428571 0.02857143 0.04285714 0.05714286 0.07142857 0.08571429 0.1 0.11428571 0.12857143 0.14285714 0.15714286 0.17142857 0.18571429 0.2 0.21428571 0.22857143 0.24285714 0.25714286 0.27142857 0.28571429 0.3 0.31428571 0.32857143 0.34285714 0.35714286 0.37142857 0.38571429 0.4 0.41428571 0.42857143 0.44285714 0.45714286 0.47142857 0.48571429 0.5 0.51428571 0.52857143 0.54285714 0.55714286 0.57142857 0.58571429 0.6 0.61428571 0.62857143 0.64285714 0.65714286 0.67142857 0.68571429 0.7 0.71428571 0.72857143 0.74285714 0.75714286 0.77142857 0.78571429 0.8 0.81428571 0.82857143 0.84285714 0.85714286 0.87142857 0.88571429 0.9 0.91428571 0.92857143 0.94285714 0.95714286 0.97142857 0.98571429 1 1 1 1 1 1
  line L6831 (268.1665, 125.8052) -> (268.1948, 125.7929) construction
  line L6832 (268.1948, 125.7929) -> (268.2518, 125.7692) construction
  line L6833 (268.2518, 125.7692) -> (268.3382, 125.736) construction
  line L6834 (268.3382, 125.736) -> (268.4549, 125.6961) construction
  line L6835 (268.4549, 125.6961) -> (268.6031, 125.6522) construction
  line L6836 (268.6031, 125.6522) -> (268.7528, 125.6127) construction
  line L6837 (268.7528, 125.6127) -> (268.9034, 125.5759) construction
  line L6838 (268.9034, 125.5759) -> (269.0546, 125.5405) construction
  line L6839 (269.0546, 125.5405) -> (269.2061, 125.506) construction
  line L6840 (269.2061, 125.506) -> (269.358, 125.4726) construction
  line L6841 (269.358, 125.4726) -> (269.5103, 125.4406) construction
  line L6842 (269.5103, 125.4406) -> (269.6632, 125.4104) construction
  line L6843 (269.6632, 125.4104) -> (269.8168, 125.3824) construction
  line L6844 (269.8168, 125.3824) -> (269.9711, 125.3565) construction
  line L6845 (269.9711, 125.3565) -> (270.126, 125.3326) construction
  line L6846 (270.126, 125.3326) -> (270.2814, 125.3103) construction
  line L6847 (270.2814, 125.3103) -> (270.4372, 125.2895) construction
  line L6848 (270.4372, 125.2895) -> (270.5934, 125.2699) construction
  line L6849 (270.5934, 125.2699) -> (270.7499, 125.2515) construction
  line L6850 (270.7499, 125.2515) -> (270.9067, 125.2342) construction
  line L6851 (270.9067, 125.2342) -> (271.0638, 125.2182) construction
  line L6852 (271.0638, 125.2182) -> (271.2213, 125.2035) construction
  line L6853 (271.2213, 125.2035) -> (271.3791, 125.1902) construction
  line L6854 (271.3791, 125.1902) -> (271.5373, 125.1782) construction
  line L6855 (271.5373, 125.1782) -> (271.6958, 125.1675) construction
  line L6856 (271.6958, 125.1675) -> (271.8546, 125.158) construction
  line L6857 (271.8546, 125.158) -> (272.0137, 125.1496) construction
  line L6858 (272.0137, 125.1496) -> (272.1731, 125.1423) construction
  line L6859 (272.1731, 125.1423) -> (272.3327, 125.1362) construction
  line L6860 (272.3327, 125.1362) -> (272.4925, 125.1311) construction
  line L6861 (272.4925, 125.1311) -> (272.6526, 125.1271) construction
  line L6862 (272.6526, 125.1271) -> (272.8129, 125.1243) construction
  line L6863 (272.8129, 125.1243) -> (272.9735, 125.1224) construction
  line L6864 (272.9735, 125.1224) -> (273.1343, 125.1217) construction
  line L6865 (273.1343, 125.1217) -> (273.2953, 125.122) construction
  line L6866 (273.2953, 125.122) -> (273.4565, 125.1234) construction
  line L6867 (273.4565, 125.1234) -> (273.6179, 125.1258) construction
  line L6868 (273.6179, 125.1258) -> (273.7795, 125.1292) construction
  line L6869 (273.7795, 125.1292) -> (273.9413, 125.1335) construction
  line L6870 (273.9413, 125.1335) -> (274.1032, 125.1389) construction
  line L6871 (274.1032, 125.1389) -> (274.2654, 125.1452) construction
  line L6872 (274.2654, 125.1452) -> (274.4277, 125.1525) construction
  line L6873 (274.4277, 125.1525) -> (274.5901, 125.1608) construction
  line L6874 (274.5901, 125.1608) -> (274.7527, 125.17) construction
  line L6875 (274.7527, 125.17) -> (274.9155, 125.1801) construction
  line L6876 (274.9155, 125.1801) -> (275.0784, 125.1912) construction
  line L6877 (275.0784, 125.1912) -> (275.2415, 125.2033) construction
  line L6878 (275.2415, 125.2033) -> (275.4047, 125.2162) construction
  line L6879 (275.4047, 125.2162) -> (275.568, 125.23) construction
  line L6880 (275.568, 125.23) -> (275.7315, 125.2448) construction
  line L6881 (275.7315, 125.2448) -> (275.8951, 125.2604) construction
  line L6882 (275.8951, 125.2604) -> (276.0588, 125.277) construction
  line L6883 (276.0588, 125.277) -> (276.2226, 125.2944) construction
  line L6884 (276.2226, 125.2944) -> (276.3865, 125.3127) construction
  line L6885 (276.3865, 125.3127) -> (276.5505, 125.3319) construction
  line L6886 (276.5505, 125.3319) -> (276.7146, 125.352) construction
  line L6887 (276.7146, 125.352) -> (276.8788, 125.3729) construction
  line L6888 (276.8788, 125.3729) -> (277.0431, 125.3946) construction
  line L6889 (277.0431, 125.3946) -> (277.2075, 125.4172) construction
  line L6890 (277.2075, 125.4172) -> (277.372, 125.4407) construction
  line L6891 (277.372, 125.4407) -> (277.5366, 125.465) construction
  line L6892 (277.5366, 125.465) -> (277.7012, 125.4902) construction
  line L6893 (277.7012, 125.4902) -> (277.866, 125.5161) construction
  line L6894 (277.866, 125.5161) -> (278.0307, 125.5429) construction
  line L6895 (278.0307, 125.5429) -> (278.1956, 125.5706) construction
  line L6896 (278.1956, 125.5706) -> (278.3605, 125.599) construction
  line L6897 (278.3605, 125.599) -> (278.5255, 125.6282) construction
  line L6898 (278.5255, 125.6282) -> (278.6905, 125.6583) construction
  line L6899 (278.6905, 125.6583) -> (278.8556, 125.6892) construction
  line L6900 (278.8556, 125.6892) -> (279.0207, 125.7208) construction
  line L6901 (279.0207, 125.7208) -> (279.1528, 125.7468) construction
  line L6902 (279.1528, 125.7468) -> (279.2519, 125.7666) construction
  line L6903 (279.2519, 125.7666) -> (279.318, 125.78) construction
  line L6904 (279.318, 125.78) -> (279.3511, 125.7868) construction
  arc A180 (225.137, 92.0377) -> (222.8136, 93.565) centre (223.1855, 91.5999) ccw
  circle A181 centre (212.132, 150) radius 2.3
  spline S92 degree 5 poles (264.6423, 181.1115) (264.6688, 181.1272) (264.7215, 181.1594) (264.7992, 181.2097) (264.9001, 181.2807) (265.0226, 181.3748) (265.1426, 181.4727) (265.2609, 181.5729) (265.3784, 181.6744) (265.4954, 181.7767) (265.6117, 181.88) (265.7271, 181.9844) (265.8414, 182.0903) (265.9544, 182.1981) (266.066, 182.3077) (266.1764, 182.419) (266.2857, 182.5316) (266.3942, 182.6455) (266.5018, 182.7603) (266.6087, 182.876) (266.7148, 182.9927) (266.8201, 183.1105) (266.9246, 183.2292) (267.0281, 183.3491) (267.1308, 183.47) (267.2327, 183.5919) (267.3337, 183.7148) (267.434, 183.8386) (267.5335, 183.9633) (267.6323, 184.0888) (267.7304, 184.2151) (267.8277, 184.3423) (267.9243, 184.4703) (268.0201, 184.5991) (268.1152, 184.7288) (268.2096, 184.8592) (268.3032, 184.9905) (268.3962, 185.1224) (268.4884, 185.2552) (268.58, 185.3886) (268.6708, 185.5228) (268.761, 185.6577) (268.8505, 185.7933) (268.9393, 185.9295) (269.0275, 186.0665) (269.1149, 186.2042) (269.2017, 186.3425) (269.2878, 186.4815) (269.3733, 186.6211) (269.4581, 186.7614) (269.5422, 186.9023) (269.6257, 187.0438) (269.7085, 187.186) (269.7907, 187.3288) (269.8723, 187.4721) (269.9532, 187.6161) (270.0334, 187.7607) (270.113, 187.9058) (270.192, 188.0515) (270.2703, 188.1978) (270.348, 188.3447) (270.4251, 188.4921) (270.5015, 188.6401) (270.5773, 188.7886) (270.6525, 188.9377) (270.727, 189.0873) (270.801, 189.2374) (270.8743, 189.3881) (270.9469, 189.5393) (271.019, 189.6909) (271.0904, 189.8431) (271.1471, 189.9653) (271.1893, 190.0572) (271.2173, 190.1185) (271.2313, 190.1492) knots 0 0 0 0 0 0 0.01428571 0.02857143 0.04285714 0.05714286 0.07142857 0.08571429 0.1 0.11428571 0.12857143 0.14285714 0.15714286 0.17142857 0.18571429 0.2 0.21428571 0.22857143 0.24285714 0.25714286 0.27142857 0.28571429 0.3 0.31428571 0.32857143 0.34285714 0.35714286 0.37142857 0.38571429 0.4 0.41428571 0.42857143 0.44285714 0.45714286 0.47142857 0.48571429 0.5 0.51428571 0.52857143 0.54285714 0.55714286 0.57142857 0.58571429 0.6 0.61428571 0.62857143 0.64285714 0.65714286 0.67142857 0.68571429 0.7 0.71428571 0.72857143 0.74285714 0.75714286 0.77142857 0.78571429 0.8 0.81428571 0.82857143 0.84285714 0.85714286 0.87142857 0.88571429 0.9 0.91428571 0.92857143 0.94285714 0.95714286 0.97142857 0.98571429 1 1 1 1 1 1
  line L6905 (264.6423, 181.1115) -> (264.6688, 181.1272) construction
  line L6906 (264.6688, 181.1272) -> (264.7215, 181.1594) construction
  line L6907 (264.7215, 181.1594) -> (264.7992, 181.2097) construction
  line L6908 (264.7992, 181.2097) -> (264.9001, 181.2807) construction
  line L6909 (264.9001, 181.2807) -> (265.0226, 181.3748) construction
  line L6910 (265.0226, 181.3748) -> (265.1426, 181.4727) construction
  line L6911 (265.1426, 181.4727) -> (265.2609, 181.5729) construction
  line L6912 (265.2609, 181.5729) -> (265.3784, 181.6744) construction
  line L6913 (265.3784, 181.6744) -> (265.4954, 181.7767) construction
  line L6914 (265.4954, 181.7767) -> (265.6117, 181.88) construction
  line L6915 (265.6117, 181.88) -> (265.7271, 181.9844) construction
  line L6916 (265.7271, 181.9844) -> (265.8414, 182.0903) construction
  line L6917 (265.8414, 182.0903) -> (265.9544, 182.1981) construction
  line L6918 (265.9544, 182.1981) -> (266.066, 182.3077) construction
  line L6919 (266.066, 182.3077) -> (266.1764, 182.419) construction
  line L6920 (266.1764, 182.419) -> (266.2857, 182.5316) construction
  line L6921 (266.2857, 182.5316) -> (266.3942, 182.6455) construction
  line L6922 (266.3942, 182.6455) -> (266.5018, 182.7603) construction
  line L6923 (266.5018, 182.7603) -> (266.6087, 182.876) construction
  line L6924 (266.6087, 182.876) -> (266.7148, 182.9927) construction
  line L6925 (266.7148, 182.9927) -> (266.8201, 183.1105) construction
  line L6926 (266.8201, 183.1105) -> (266.9246, 183.2292) construction